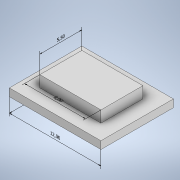
# Autodesk Inventor part: Button
Saved by Autodesk Inventor 2020.1 (Build 241239000, 239)
## iProperties
Created: 2020-05-23
Part Number: Button
Material: Generic
Document SubType Name: Modeling
Designer: super
Density: 1 g/cm^3
Appearance: Default
Author: super
Autodesk Inventor part; units mm, degrees
ref_plane "YZ Plane" through (0, 0, 0) normal (1, 0, 0) x (0, 1, 0)
ref_plane "XZ Plane" through (0, 0, 0) normal (0, 1, 0) x (-1, 0, 0)
ref_plane "XY Plane" through (0, 0, 0) normal (0, 0, 1) x (1, 0, 0)
sketch "Sketch1" plane through (0, 0, 0) normal (0, 1, 0) x (-1, 0, 0)
  line L0 (0, 0) -> (-8, 0)
  line L1 (-8, 0) -> (-8, 6)
  line L2 (-8, 6) -> (0, 6)
  line L3 (0, 6) -> (0, 0)
  dimension "d0" = 8
  dimension "d1" = 6
  constraints: 8 end point, 2 parallel, 1 horizontal, 1 perpendicular
  measures "d0" distance of L1.end L2.end
  measures "d1" distance of L0.end L1.end
extrude "Extrusion1" add sketch "Sketch1" along normal blind 1.5
sketch "Sketch2" plane through (0, 0, 0) normal (0, -1, 0) x (1, 0, 0)
  line L0 (8, 0) -> (0, 0) projected
  line L1 (8, 0) -> (0, 0)
  line L2 (8, 6) -> (8, 0) projected
  line L3 (0, 6) -> (8, 6)
  line L4 (8, 6) -> (8, 0)
  line L5 (0, 5.5) -> (8, 5.5)
  line L6 (0, 5.5) -> (0, 6)
  line L7 (0, 6) -> (8, 6) projected
  line L8 (8, 6) -> (8, 5.5)
  line L9 (8, 6) -> (0, 6)
  dimension "d4" = 5.5
  constraints: 14 end point, 3 perpendicular, 1 horizontal, 1 parallel, 1 point on line
  measures "d4" distance of L0.end L5.start
extrude "Extrusion2" cut sketch "Sketch2" against normal blind 10
sketch "Sketch3" plane through (0, 0, 0) normal (0, -1, 0) x (1, 0, 0)
  point P0 (0, 0)
sketch "Sketch4" plane through (0, 0, 0) normal (0, -1, 0) x (1, 0, 0)
  line L0 (8, 0) -> (0, 0) projected
  line L1 (0, -2) -> (10, -2)
  line L2 (10, -2) -> (10, 7.5)
  line L3 (10, 7.5) -> (-2, 7.5)
  line L4 (-2, 7.5) -> (-2, -2)
  line L5 (-2, -2) -> (0, -2)
  dimension "d7" = 2
  dimension "d8" = 10
  dimension "d9" = 9.5
  dimension "d10" = 12
  constraints: 10 end point, 4 perpendicular, 1 point on line
  measures "d7" distance of L0.end L1.start
  measures "d8" distance of L1.start L1.end
  measures "d9" distance of L1.end L2.end
  measures "d10" distance of L2.end L3.end
extrude "Extrusion3" add sketch "Sketch4" along normal blind 1
body "Solid1"
